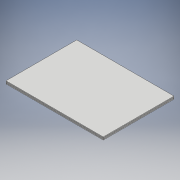
# Autodesk Inventor part: Game_TurmoilCard
Saved by Autodesk Inventor 2018 (Build 220112000, 112)
## iProperties
Created: 2021-04-21
Part Number: Game_TurmoilCard
Material: Generic
Document SubType Name: Modeling
Designer: Bradley
Density: 1 g/cm^3
Appearance: Default
Author: Bradley
Autodesk Inventor part; units mm, degrees
ref_plane "YZ Plane" through (0, 0, 0) normal (1, 0, 0) x (0, 1, 0)
ref_plane "XZ Plane" through (0, 0, 0) normal (0, 1, 0) x (-1, 0, 0)
ref_plane "XY Plane" through (0, 0, 0) normal (0, 0, 1) x (1, 0, 0)
sketch "Sketch1" plane through (0, 0, 0) normal (0, 0, 1) x (1, 0, 0)
  line L0 (-110, -80) -> (110, -80)
  line L1 (110, -80) -> (110, 80)
  line L2 (110, 80) -> (-110, 80)
  line L3 (-110, 80) -> (-110, -80)
  line L4 (-110, -80) -> (110, 80) construction
  line L5 (110, -80) -> (-110, 80) construction
  point P0 (0, 0)
  dimension "d0" = 220
  dimension "d1" = 160
  constraints: 12 end point, 2 midpoint, 2 parallel, 1 horizontal, 1 perpendicular
  measures "d0" distance of L2.end L1.end
  measures "d1" distance of L1.end L0.end
extrude "Extrusion1" add sketch "Sketch1" along normal mid plane 2
pattern_linear "Rectangular Pattern1" count 3 spacing 2.1 along (0, 0, 1) of "Extrusion1"
body "Solid1"
